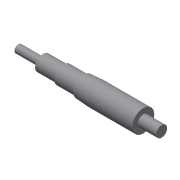
# Autodesk Inventor part: 00_Micrometer
Saved by Autodesk Inventor 2019 (Build 230136000, 136)
## iProperties
Created: 2019-11-02
Part Number: 00_Micrometer
Material: Generic
Document SubType Name: Modeling
Designer: diederichbenedict
Density: 1 g/cm^3
Appearance: Default
Author: diederichbenedict
Autodesk Inventor part; units mm, degrees
ref_plane "YZ Plane" through (0, 0, 0) normal (1, 0, 0) x (0, 1, 0)
ref_plane "XZ Plane" through (0, 0, 0) normal (0, 1, 0) x (-1, 0, 0)
ref_plane "XY Plane" through (0, 0, 0) normal (0, 0, 1) x (1, 0, 0)
sketch "Sketch1" plane through (0, 0, 0) normal (0, 0, 1) x (1, 0, 0)
  line L0 (0, 0) -> (20, 0)
  line L1 (20, 0) -> (20, 3.2)
  line L2 (20, 3.2) -> (0, 3.2)
  line L3 (0, 3.2) -> (0, 0)
  line L4 (20, 0) -> (36.65, 0)
  line L5 (36.65, 0) -> (36.65, 6.335)
  line L6 (36.65, 6.335) -> (20, 6.335)
  line L7 (20, 6.335) -> (20, 0)
  line L8 (36.65, 0) -> (53.17, 0)
  line L9 (53.17, 0) -> (53.17, 7.26)
  line L10 (53.17, 7.26) -> (36.65, 7.26)
  line L11 (36.65, 7.26) -> (36.65, 0)
  line L12 (53.17, 0) -> (102.07, 0)
  line L13 (102.07, 0) -> (102.07, 9)
  line L14 (102.07, 9) -> (64.2031, 9)
  line L15 (53.17, 9) -> (53.17, 0)
  line L16 (102.07, 0) -> (117.1074, 0)
  line L17 (117.1074, 0) -> (117.1074, 4.5)
  line L18 (117.1074, 4.5) -> (102.07, 4.5)
  line L19 (102.07, 4.5) -> (102.07, 0)
  line L20 (53.17, 8.2611) -> (64.2031, 9)
  dimension "d0" = 20
  dimension "d1" = 3.2
  dimension "d2" = 16.65
  dimension "d3" = 6.335
  dimension "d4" = 16.52
  dimension "d5" = 7.26
  dimension "d6" = 48.9
  dimension "d7" = 9
  constraints: 42 end point, 10 parallel, 5 horizontal, 5 perpendicular, 1 point on line
  measures "d0" distance of L2.end L1.end
  measures "d1" distance of L1.end L0.end
  measures "d2" distance of L6.end L5.end
  measures "d3" distance of L5.end L4.end
  measures "d4" distance of L10.end L9.end
  measures "d5" distance of L9.end L8.end
  measures "d6" distance of L15.start L13.end
  measures "d7" distance of L13.end L12.end
revolve "Revolution1" add sketch "Sketch1" angle 360 about axis through (53.17, 0, 0) along (1, 0, 0)
body "Solid1"
